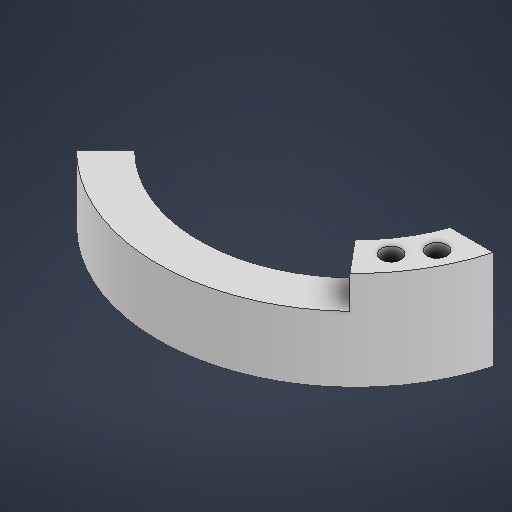
# Autodesk Inventor part: Part4
Saved by Autodesk Inventor 2026.1 (Build 301233020, 233B)
## iProperties
Created: 2025-10-15
Part Number: Part4
Material: Generic
Document SubType Name: Modeling
Designer: Desktop
Density: 1 g/cm^3
Appearance: Default
Author: Desktop
Autodesk Inventor part; units mm, degrees
ref_plane "YZ Plane" through (0, 0, 0) normal (1, 0, 0) x (0, 1, 0)
ref_plane "XZ Plane" through (0, 0, 0) normal (0, 1, 0) x (-1, 0, 0)
ref_plane "XY Plane" through (0, 0, 0) normal (0, 0, 1) x (1, 0, 0)
sketch "Sketch1" plane through (0, 0, 0) normal (0, 1, 0) x (-1, 0, 0)
  line L0 (89.9885, -104.2218) -> (68.0145, -104.2218) construction
  line L1 (68.0145, -104.2218) -> (61.4656, -104.2218)
  circle A0 centre (66.0145, -100.2218) radius 1.5
  circle A1 centre (68.5368, -96.2218) radius 1.5
  line L2 (107.1822, -95.395) -> (90.3884, -112.1888)
  arc A2 (107.1822, -95.395) -> (68.0145, -104.2218) centre (90.3884, -112.1888) ccw
  arc A3 (111.6013, -90.9754) -> (61.4656, -104.2218) centre (90.3884, -112.1888) ccw
  line L3 (111.6013, -90.9754) -> (107.1822, -95.395)
  point P0 (0, 0)
  point P1 (72.3101, -96.7863)
  point P2 (68.5146, -91.6574)
  point P3 (64.74, -104.2218)
  point P4 (70.4123, -94.2218)
  dimension "d0" = 47.5
  dimension "d1" = 60
  dimension "d2" = 115.4
  dimension "d3" = 45
  dimension "d4" = 2
  dimension "d5" = 4
  dimension "d6" = 8
  dimension "d7" = 10
  constraints: 8 end point, 6 point on circle, 4 centre point, 1 coincident, 1 collinear, 1 horizontal, 1 midpoint
  measures "d0" diameter of A2
  measures "d1" diameter of A3
  measures "d3" angle of L2 L0
  measures "d4" horizontal distance of A0.centre L0.end
  measures "d5" distance from line of A0.centre L1
  measures "d6" distance from line of A1.centre L1
  measures "d7" vertical distance of point (64.74, -104.222) point (70.412, -94.222)
extrude "Extrusion1" add sketch "Sketch1" along normal blind 10 contours L1 A3 L3 A2 | A0 | A1
sketch "Sketch2" plane through (0, 10, 0) normal (0, 1, 0) x (1, 0, 0)
  circle A0 centre (-66.0145, 100.2218) radius 1.5
  circle A1 centre (-69.0145, 96.2218) radius 1.5
  line L0 (-61.4656, 104.2218) -> (-68.0145, 104.2218) projected
  arc A2 (-107.1822, 95.395) -> (-68.0145, 104.2218) centre (-90.3884, 112.1888) ccw projected
  line L1 (-73.6317, 95.3579) -> (-69.6037, 90.5555)
  arc A3 (-111.6013, 90.9754) -> (-61.4656, 104.2218) centre (-90.3884, 112.1888) ccw projected
  point P0 (0, 0)
  dimension "d10" = 3
  dimension "d11" = 3
  dimension "d12" = 4
  dimension "d13" = 8
  dimension "d14" = 2
  dimension "d16" = 50.012
  dimension "d17" = 10
  constraints: 2 centre point, 2 end point, 2 point on circle
  measures "d10" diameter of A0
  measures "d11" diameter of A1
  measures "d12" distance from line of L0 A0.centre
  measures "d13" distance from line of L0 A1.centre
  measures "d14" horizontal distance of A0.centre L0.end
  measures "d16" angle of L0 L1
  measures "d17" distance from line of L0.end L1
extrude "Extrusion2" add sketch "Sketch2" along normal blind 5
body "Solid1"
